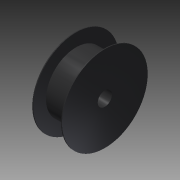
# Autodesk Inventor part: rolka_filamentu
Saved by Autodesk Inventor 2013 (Build 170138000, 138)
## iProperties
Created: 2014-04-26
Part Number: rolka_filamentu
Material: Generic
Document SubType Name: Modeling
Designer: Masta
Density: 1 g/cm^3
Author: Masta
Autodesk Inventor part; units mm, degrees
ref_plane "YZ Plane" through (0, 0, 0) normal (1, 0, 0) x (0, 1, 0)
ref_plane "XZ Plane" through (0, 0, 0) normal (0, 1, 0) x (-1, 0, 0)
ref_plane "XY Plane" through (0, 0, 0) normal (0, 0, 1) x (1, 0, 0)
sketch "Sketch1" plane through (0, 0, 0) normal (0, 0, 1) x (1, 0, 0)
  line L0 (0, 0) -> (52, 0)
  line L1 (52, 0) -> (52, 150)
  line L2 (52, 150) -> (49, 150)
  line L3 (49, 150) -> (49, 105)
  line L4 (49, 105) -> (0, 105)
  line L5 (0, 105) -> (0, 0)
  line L6 (0, 25) -> (52, 25)
  dimension "d0" = 52
  dimension "d1" = 150
  dimension "d2" = 3
  dimension "d3" = 25
  dimension "d4" = 105
  constraints: 14 end point, 3 parallel, 3 perpendicular, 2 point on line, 1 horizontal
  measures "d0" distance of L0.start L0.end
  measures "d1" distance of L0.end L1.end
  measures "d2" distance of L1.end L2.end
  measures "d3" distance between parallel lines of L0 L6
  measures "d4" distance between parallel lines of L0 L4
revolve "Revolution1" add sketch "Sketch1" angle 360 about axis through (0, 0, 0) along (1, 0, 0) contours L5 L4 L3 L2 L1 L6
mirror "Mirror1" about plane through (0, 65, 0) normal (-1, 0, 0) of "Revolution1"
body "Solid1"
